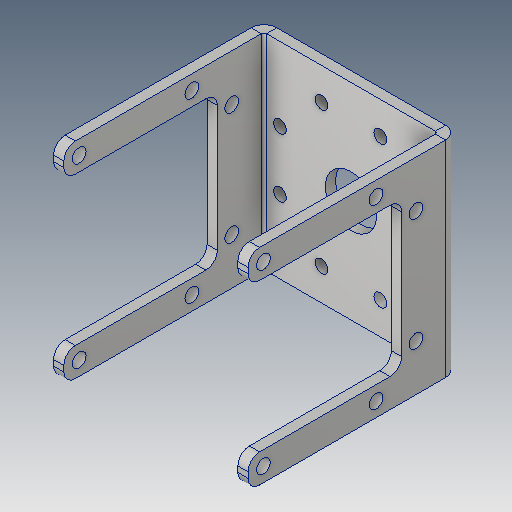
# Autodesk Inventor part: 조인트4연결부
Saved by Autodesk Inventor 2020.5 (Build 245400000, 400)
## iProperties
Created: 2021-07-12
Part Number: 조인트4연결부
Material: 알루미늄 6061
Document SubType Name: Sheet Metal
Designer: user
Density: 2.7 g/cm^3
Sheet Metal Rule: 기본값_mm
Appearance: 알루미늄 - 평지
Mass: 14.5185 g
Surface Area: 66.0658 cm^2
Volume: 5.37723 cm^3
Flat Pattern Width: 4.02 cm
Flat Pattern Length: 11.4535 cm
Flat Pattern Area: 46.0432 cm^2
Sheet Metal Width: 40.200 mm
Sheet Metal Length: 114.535 mm
Sheet Metal Area: 4604.323 mm^2
Author: user
Autodesk Inventor part; units mm, degrees
ref_plane "YZ Plane" through (0, 0, 0) normal (1, 0, 0) x (0, 1, 0)
ref_plane "XZ Plane" through (0, 0, 0) normal (0, 1, 0) x (-1, 0, 0)
ref_plane "XY Plane" through (0, 0, 0) normal (0, 0, 1) x (1, 0, 0)
sketch "스케치1" plane through (0, 0, 0) normal (0, 0, 1) x (1, 0, 0)
  line L0 (-17, 20.1) -> (17, 20.1)
  line L1 (17, 20.1) -> (17, -20.1)
  line L2 (17, -20.1) -> (-17, -20.1)
  line L3 (-17, -20.1) -> (-17, 20.1)
  point P0 (0, 0)
  dimension "d0" = 34
  dimension "d1" = 17
  dimension "d2" = 40.2
  dimension "d3" = 20.1
  constraints: 8 end point, 2 parallel, 1 horizontal, 1 perpendicular
  measures "d0" distance of L1.end L2.end
  measures "d1" distance from line of L3 point (0, 0)
  measures "d2" distance between parallel lines of L2 L0
  measures "d3" distance from line of point (0, 0) L0
extrude "돌출1" add sketch "스케치1" along normal blind 2
sketch "스케치2" plane through (17, 20.1, 2) normal (1, 0, 0) x (0, 1, 0)
  line L0 (-40.2, 0) -> (0, 0)
  line L1 (0, 0) -> (0, 39.1)
  line L2 (0, 39.1) -> (-40.2, 39.1)
  line L3 (-40.2, 39.1) -> (-40.2, 0)
  constraints: 4 end point, 4 other
edge flange "플랜지1" height 41.1 angle 90 thickness 2 bend radius 0.5 thickness toward (1, 0, 0) relief tear relief width 2 relief depth 1 corner gap 2 corner form 0 edges at (17, 0, 2) (-17, 0, 2) wall of the first edge with corners at (17, -20.1, 2) (17, 20.1, 2) (17, 20.1, 41.1) (17, -20.1, 41.1)
bend "절곡부1"
corner "구석1"
sketch "스케치3" plane through (-19, -20.1, 41.1) normal (-1, 0, 0) x (0, 0, 1)
  line L0 (-38.6, 40.2) -> (-38.6, 0) projected
  line L1 (-41.1, 40.2) -> (-38.6, 40.2) projected
  line L2 (-41.1, 0) -> (-41.1, 40.2) projected
  line L3 (-38.6, 0) -> (-41.1, 0) projected
  line L4 (-39.1, 40.2) -> (-41.1, 40.2) projected
  line L5 (-39.1, 40.2) -> (-38.1, 40.2)
  line L6 (-38.1, 0) -> (-39.1, 0)
  line L7 (-30, 11.85) -> (-30, 28.35)
  line L8 (-23.75, 34.6) -> (23.25, 34.6)
  arc A0 (24.25, 33.6) -> (23.25, 34.6) centre (23.25, 33.6) ccw
  line L9 (24.25, 33.6) -> (24.25, 31.6)
  arc A1 (24.25, 31.6) -> (26.5, 29.35) centre (26.5, 31.6) ccw
  line L10 (26.5, 29.35) -> (27.25, 29.35)
  line L11 (29.5, 35.1) -> (29.5, 31.6)
  line L12 (23.5, 40.2) -> (29.5, 35.1)
  line L13 (-29.6, 40.2) -> (23.5, 40.2)
  line L14 (-35.6, 35.1) -> (-29.6, 40.2)
  line L15 (-35.6, 5.1) -> (-35.6, 35.1)
  line L16 (-29.6, 0) -> (-35.6, 5.1)
  line L17 (23.5, 0) -> (-29.6, 0)
  line L18 (29.5, 5.1) -> (23.5, 0)
  line L19 (29.5, 8.6) -> (29.5, 5.1)
  line L20 (27.25, 10.85) -> (26.5, 10.85)
  arc A2 (26.5, 10.85) -> (24.25, 8.6) centre (26.5, 8.6) ccw
  line L21 (24.25, 8.6) -> (24.25, 6.6)
  arc A3 (23.25, 5.6) -> (24.25, 6.6) centre (23.25, 6.6) ccw
  line L22 (23.25, 5.6) -> (-23.75, 5.6)
  circle A4 centre (19, 2.8) radius 1.35
  circle A5 centre (-3, 2.8) radius 1.35
  circle A6 centre (-32.8, 9.1) radius 1.35
  circle A7 centre (19, 37.4) radius 1.35
  circle A8 centre (-3, 37.4) radius 1.35
  circle A9 centre (-32.8, 31.1) radius 1.35
  circle A10 centre (-25, 2.8) radius 1.35
  circle A11 centre (-25, 37.4) radius 1.35
  line L23 (-38.6, 0) -> (-38.6, 40.2) projected
  line L24 (-38.6, 40.2) -> (0, 40.2) projected
  line L25 (0, 40.2) -> (0, 0) projected
  line L26 (-23.75, 34.6) -> (-27.75, 34.6)
  line L27 (-30, 28.35) -> (-30, 32.35)
  line L28 (-30, 11.85) -> (-30, 7.85)
  line L29 (-23.75, 5.6) -> (-27.75, 5.6)
  arc A12 (-27.75, 34.6) -> (-30, 32.35) centre (-27.75, 32.35) ccw
  arc A13 (-30, 7.85) -> (-27.75, 5.6) centre (-27.75, 7.85) ccw
  arc A14 (29.5, 8.6) -> (27.25, 10.85) centre (27.25, 8.6) ccw
  arc A15 (27.25, 29.35) -> (29.5, 31.6) centre (27.25, 31.6) ccw
  line L30 (-32.8, 31.1) -> (-38.6, 31.1)
  line L31 (-38.6, 40.2) -> (-38.6, 0) projected
  point P0 (-41.1, 20.1)
  point P1 (15, 20.1)
  point P2 (0, 5.6)
  point P3 (0, 34.6)
  dimension "d18" = 40.2
  dimension "d93" = 2.25
  dimension "d96" = 5.8
  constraints: 46 end point, 16 centre point, 16 point on circle, 8 tangent, 3 equal radius, 3 horizontal, 2 vertical, 1 parallel, 1 perpendicular, 1 point on line
  measures "d18" distance of L5.end L6.start
  measures "d93" radius of A12
  measures "d96" distance of L30.start L30.end
extrude "돌출2" cut sketch "스케치3" against normal up to surface (38 mm away) contours L25 L22 L29 A13 L28 L7 L27 A12 L26 L8 | A5 | A6 | A8 | A9 | A10 | A11
sketch "스케치6" plane through (0, 0, 0) normal (0, 0, -1) x (-1, 0, 0)
  circle A0 centre (0, 0) radius 14 construction
  line L0 (0, 0) -> (-5.7403, 13.8582)
  line L1 (0, 0) -> (15, 0) construction
  circle A1 centre (-5.7403, 13.8582) radius 1.25
  circle A2 centre (-13.8582, 5.7403) radius 1.25
  circle A3 centre (-13.8582, -5.7403) radius 1.25
  circle A4 centre (-5.7403, -13.8582) radius 1.25
  circle A5 centre (5.7403, -13.8582) radius 1.25
  circle A6 centre (13.8582, -5.7403) radius 1.25
  circle A7 centre (13.8582, 5.7403) radius 1.25
  circle A8 centre (5.7403, 13.8582) radius 1.25
  circle A9 centre (0, 0) radius 5
  dimension "d108" = 28
  dimension "d109" = 15
  dimension "d110" = 112.5
  dimension "d111" = 2.5
  dimension "d112" = 360
  dimension "d113" = 10
  constraints: 10 centre point, 4 end point, 3 coincident, 1 equal length, 1 horizontal, 17 other
  measures "d108" diameter of A0
  measures "d109" distance of L0.start L0.end
  measures "d110" angle of L1 L0
  measures "d111" diameter of A1
  measures "d113" diameter of A9
extrude "돌출8" cut sketch "스케치6" against normal up to surface (2 mm away)
fillet "모깎기4" radius 2.25 8 edges at (-18, 20.1, 41.1) (-18, 14.5, 41.1) (18, 20.1, 41.1) (18, 14.5, 41.1) (18, -14.5, 41.1) (18, -20.1, 41.1) (-18, -14.5, 41.1) (-18, -20.1, 41.1)
equation "\"d1\" = 0.5 * d0"
equation "\"d3\" = 0.5 * d2"
equation "\"d7\" = BendReliefWidth"
equation "\"d8\" = BendReliefDepth"
equation "\"d9\" = MinimumRemnant"
equation "\"d10\" = TransitionRadius"
equation "\"d14\" = CornerReliefSize"
equation "\"TransitionRadius\" = BendRadius"
equation "\"BendReliefWidth\" = 2"
equation "\"BendReliefDepth\" = 1"
equation "\"MinimumRemnant\" = 4"
equation "\"CornerReliefSize\" = 8"
equation "\"BendRadius\" = 2"
